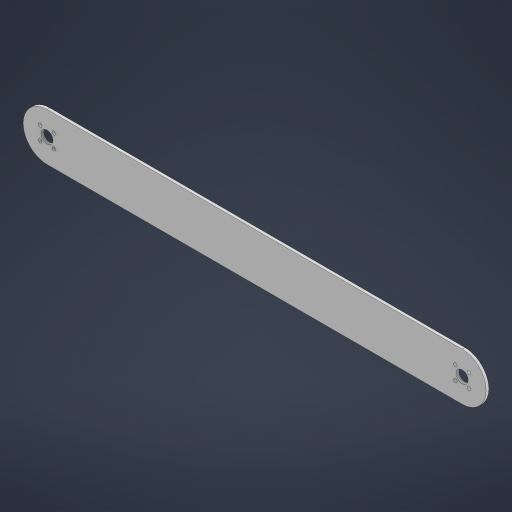
# Autodesk Inventor part: SecondStageArmBar
Saved by Autodesk Inventor 2024 (Build 280153000, 153)
## iProperties
Created: 2023-11-24
Part Number: SecondStageArmBar
Material: Generic
Document SubType Name: Modeling
Designer: avsar
Density: 1 g/cm^3
Appearance: Default
Author: avsar
Autodesk Inventor part; units mm, degrees
ref_plane "YZ Plane" through (0, 0, 0) normal (1, 0, 0) x (0, 1, 0)
ref_plane "XZ Plane" through (0, 0, 0) normal (0, 1, 0) x (-1, 0, 0)
ref_plane "XY Plane" through (0, 0, 0) normal (0, 0, 1) x (1, 0, 0)
sketch "Sketch1" plane through (0, 0, 0) normal (0, 0, 1) x (1, 0, 0)
  line L0 (-244, -28) -> (244, -28)
  line L1 (272, 0) -> (272, 0)
  line L2 (244, 28) -> (-244, 28)
  line L3 (-272, 0) -> (-272, 0)
  line L4 (-272, -28) -> (272, 28) construction
  line L5 (272, -28) -> (-272, 28) construction
  arc A0 (272, 0) -> (244, 28) centre (244, 0) ccw
  arc A1 (244, -28) -> (272, 0) centre (244, 0) ccw
  arc A2 (-272, 0) -> (-244, -28) centre (-244, 0) ccw
  arc A3 (-244, 28) -> (-272, 0) centre (-244, 0) ccw
  circle A4 centre (244, 0) radius 7
  circle A5 centre (-244, 0) radius 7
  circle A6 centre (-252, 8) radius 2
  circle A7 centre (-252, -8) radius 2
  circle A8 centre (-236, -8) radius 2
  circle A9 centre (-236, 8) radius 2
  circle A10 centre (252, 8) radius 2
  circle A11 centre (236, 8) radius 2
  circle A12 centre (236, -8) radius 2
  circle A13 centre (252, -8) radius 2
  point P0 (0, 0)
  point P1 (-272, 0)
  dimension "d0" = 544
  dimension "d1" = 56
  dimension "d2" = 28
  dimension "d3" = 28
  dimension "d4" = 28
  dimension "d5" = 14
  dimension "d6" = 14
  dimension "d9" = 4
  dimension "d10" = 8
  dimension "d11" = 8
  dimension "d14" = 360
  dimension "d16" = 4
  dimension "d17" = 8
  dimension "d18" = 8
  dimension "d21" = 360
  constraints: 14 centre point, 12 end point, 8 point on circle, 8 point on line, 8 tangent, 2 coincident, 2 midpoint, 2 parallel, 1 concentric, 1 horizontal, 1 perpendicular, 18 other
  measures "d0" distance of L5.end L4.end
  measures "d1" distance of L4.end L5.start
  measures "d2" radius of A0
  measures "d3" radius of A1
  measures "d4" radius of A2
  measures "d5" diameter of A4
  measures "d6" diameter of A5
  measures "d9" diameter of A6
  measures "d10" horizontal distance of A6.centre A2.centre
  measures "d11" horizontal distance of A5.centre A6.centre
  measures "d16" diameter of A10
  measures "d17" horizontal distance of A0.centre A10.centre
  measures "d18" horizontal distance of A0.centre A10.centre
extrude "Extrusion1" add sketch "Sketch1" along normal mid plane 3.175
equation "\"d2\" = 0.5 * d1"
equation "\"d3\" = d2"
equation "\"d4\" = d2"
body "Solid1"
